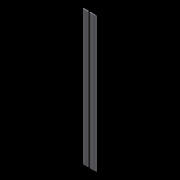
# Autodesk Inventor part: 3d_LM - Bottom Wire - Phantom
Saved by Autodesk Inventor 2018.3 (Build 223284000, 284)
## iProperties
Category: 0
Created: 2026-02-16
Part Number: 3d_LM - Bottom Wire - Phantom
Material: Genérico
Document SubType Name: Modeling
Designer: aca6
Density: 1 g/cm^3
Appearance: Valor por defecto
Manufacturer-1: {"Link": "", "Name": "\nEmbention Sistemas Inteligentes S.A.", "PartNumber": "3d_LM - Bottom Wire", "partner_id": false}
Manufacturer-2: {"Link": "", "Name": "", "PartNumber": "", "partner_id": false}
Manufacturer-3: {"Link": "", "Name": "", "PartNumber": "", "partner_id": false}
Manufacturer-4: {"Link": "", "Name": "", "PartNumber": "", "partner_id": false}
Manufacturer-5: {"Link": "", "Name": "", "PartNumber": "", "partner_id": false}
Provider-1: {"Link": "", "Name": "", "PartNumber": "", "partner_id": false}
Provider-2: {"Link": "", "Name": "", "PartNumber": "", "partner_id": false}
Provider-3: {"Link": "", "Name": "", "PartNumber": "", "partner_id": false}
Provider-4: {"Link": "", "Name": "", "PartNumber": "", "partner_id": false}
Provider-5: {"Link": "", "Name": "", "PartNumber": "", "partner_id": false}
odoo_id: 22898
odoo_internal_code: P015263
odoo_model: product.product
odoo_x2o_application_version: 12.0.4.20
odoo_d2o_version: 12.0.1.6.0
Author: aca6
Autodesk Inventor part; units mm, degrees
ref_plane "YZ Plane" through (0, 0, 0) normal (1, 0, 0) x (0, 1, 0)
ref_plane "XZ Plane" through (0, 0, 0) normal (0, 1, 0) x (-1, 0, 0)
sketch "Sketch1" plane through (0, 0, 0) normal (0, 0, 1) x (1, 0, 0)
  line L0 (34.8824, 2.8037) -> (34.8824, -2.1963) projected
  line L1 (28.8824, 2.8037) -> (34.8824, 2.8037) projected
  line L2 (28.8824, 2.6037) -> (28.8824, 2.8037) projected
  line L3 (22.8824, 2.6037) -> (28.8824, 2.6037) projected
  arc A0 (21.1274, 2.6037) -> (22.8824, 2.6037) centre (22.0049, 2.8037) ccw projected
  line L4 (20.1824, 2.6037) -> (21.1274, 2.6037) projected
  arc A1 (18.4274, 2.6037) -> (20.1824, 2.6037) centre (19.3049, 2.8037) ccw projected
  line L5 (17.2951, 2.6037) -> (18.4274, 2.6037) projected
  arc A2 (13.2146, 2.6037) -> (17.2951, 2.6037) centre (15.2549, 2.8037) ccw projected
  line L6 (12.7951, 2.6037) -> (13.2146, 2.6037) projected
  arc A3 (8.7146, 2.6037) -> (12.7951, 2.6037) centre (10.7549, 2.8037) ccw projected
  line L7 (8.2951, 2.6037) -> (8.7146, 2.6037) projected
  arc A4 (4.2146, 2.6037) -> (8.2951, 2.6037) centre (6.2549, 2.8037) ccw projected
  line L8 (3.7951, 2.6037) -> (4.2146, 2.6037) projected
  arc A5 (-0.2854, 2.6037) -> (3.7951, 2.6037) centre (1.7549, 2.8037) ccw projected
  line L9 (-5.2049, 2.6037) -> (-0.2854, 2.6037) projected
  arc A6 (-9.2854, 2.6037) -> (-5.2049, 2.6037) centre (-7.2451, 2.8037) ccw projected
  line L10 (-9.7049, 2.6037) -> (-9.2854, 2.6037) projected
  arc A7 (-13.7854, 2.6037) -> (-9.7049, 2.6037) centre (-11.7451, 2.8037) ccw projected
  line L11 (-14.2049, 2.6037) -> (-13.7854, 2.6037) projected
  arc A8 (-18.2854, 2.6037) -> (-14.2049, 2.6037) centre (-16.2451, 2.8037) ccw projected
  line L12 (-18.7049, 2.6037) -> (-18.2854, 2.6037) projected
  arc A9 (-22.7854, 2.6037) -> (-18.7049, 2.6037) centre (-20.7451, 2.8037) ccw projected
  line L13 (-28.7854, 2.6037) -> (-22.7854, 2.6037) projected
  line L14 (-28.7854, 2.8037) -> (-28.7854, 2.6037) projected
  line L15 (-34.7854, 2.8037) -> (-28.7854, 2.8037) projected
  line L16 (-34.7854, -2.1963) -> (-34.7854, 2.8037) projected
  line L17 (34.8824, -2.1963) -> (-34.7854, -2.1963) projected
  line L18 (34.8824, 2.8037) -> (34.8824, 7.8037) projected
  line L19 (34.8824, 7.8037) -> (-34.7854, 7.8037) projected
  line L20 (-34.7854, 7.8037) -> (-34.7854, 2.8037) projected
  line L21 (-34.7854, 2.8037) -> (-28.7854, 2.8037) projected
  line L22 (-28.7854, 2.8037) -> (-28.7854, 3.0037) projected
  line L23 (-28.7854, 3.0037) -> (-22.7854, 3.0037) projected
  arc A10 (-18.7049, 3.0037) -> (-22.7854, 3.0037) centre (-20.7451, 2.8037) ccw projected
  line L24 (-18.7049, 3.0037) -> (-18.2854, 3.0037) projected
  arc A11 (-14.2049, 3.0037) -> (-18.2854, 3.0037) centre (-16.2451, 2.8037) ccw projected
  line L25 (-14.2049, 3.0037) -> (-13.7854, 3.0037) projected
  arc A12 (-9.7049, 3.0037) -> (-13.7854, 3.0037) centre (-11.7451, 2.8037) ccw projected
  line L26 (-9.7049, 3.0037) -> (-9.2854, 3.0037) projected
  arc A13 (-5.2049, 3.0037) -> (-9.2854, 3.0037) centre (-7.2451, 2.8037) ccw projected
  line L27 (-5.2049, 3.0037) -> (-0.2854, 3.0037) projected
  arc A14 (3.7951, 3.0037) -> (-0.2854, 3.0037) centre (1.7549, 2.8037) ccw projected
  line L28 (3.7951, 3.0037) -> (4.2146, 3.0037) projected
  arc A15 (8.2951, 3.0037) -> (4.2146, 3.0037) centre (6.2549, 2.8037) ccw projected
  line L29 (8.2951, 3.0037) -> (8.7146, 3.0037) projected
  arc A16 (12.7951, 3.0037) -> (8.7146, 3.0037) centre (10.7549, 2.8037) ccw projected
  line L30 (12.7951, 3.0037) -> (13.2146, 3.0037) projected
  arc A17 (17.2951, 3.0037) -> (13.2146, 3.0037) centre (15.2549, 2.8037) ccw projected
  line L31 (17.2951, 3.0037) -> (18.4274, 3.0037) projected
  arc A18 (20.1824, 3.0037) -> (18.4274, 3.0037) centre (19.3049, 2.8037) ccw projected
  line L32 (20.1824, 3.0037) -> (21.1274, 3.0037) projected
  arc A19 (22.8824, 3.0037) -> (21.1274, 3.0037) centre (22.0049, 2.8037) ccw projected
  line L33 (22.8824, 3.0037) -> (28.8824, 3.0037) projected
  line L34 (28.8824, 3.0037) -> (28.8824, 2.8037) projected
  line L35 (28.8824, 2.8037) -> (34.8824, 2.8037) projected
  arc A20 (21.1274, 2.6037) -> (21.1274, 3.0037) centre (22.0049, 2.8037) ccw
  arc A21 (-18.7049, 3.0037) -> (-18.7049, 2.6037) centre (-20.7451, 2.8037) ccw
  arc A22 (3.7951, 3.0037) -> (3.7951, 2.6037) centre (1.7549, 2.8037) ccw
  arc A23 (-9.2854, 2.6037) -> (-9.2854, 3.0037) centre (-7.2451, 2.8037) ccw
  point P0 (0, 0)
  constraints: 8 end point, 8 point on circle, 4 centre point, 4 coincident, 4 concentric
ref_plane "Work Plane1" through (-34.7854, -2.1963, -450) normal (0, 0, -1) x (0, 1, 0)
extrude "Extrusion1" add sketch "Sketch1" against normal up to surface (450 mm away) contours A0 L4 A1 L5 A2 L6 A3 L7 A4 L8 A5 A22 A14 L28 A15 L29 A16 L30 A17 L31 A18 L32 A19 A20 | A21 A10 L24 A11 L25 A12 L26 A13 A23 A6 L10 A7 L11 A8 L12 A9
body "Solid1"
